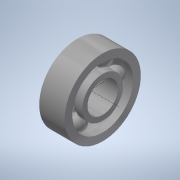
# Autodesk Inventor part: Ball bearing 15mm
Saved by Autodesk Inventor 2021 (Build 250183000, 183)
## iProperties
Manager: Pierloot J.
Company: Emmaüs Bovenbouw Aalter
Created: 2015-08-18
Part Number: Ball bearing 15mm
Material: S235
Catalog Web Link: http://emmausbovenbouw.op-weg.be/
Vendor: Emmaüsinstituut Bovenbouw Aalter
Document SubType Name: Modeling
Designer: Pierlootj
Engineer: Pierloot J.
Manufacturer: Standard
Standards Organization: Custom
Density: 7.86 g/cm^3
Appearance: Steel
Title: Algemene titel
Subject: Specifieke titel
Author: Pierlootj
Keywords: Ruwe Ø xxxxx
Comments: Opmerking
Autodesk Inventor part; units mm, degrees
ref_plane "YZ Plane" through (0, 0, 0) normal (1, 0, 0) x (0, 1, 0)
ref_plane "XZ Plane" through (0, 0, 0) normal (0, 1, 0) x (-1, 0, 0)
ref_plane "XY Plane" through (0, 0, 0) normal (0, 0, 1) x (1, 0, 0)
sketch "Sketch1" plane through (0, 0, 0) normal (0, 0, 1) x (1, 0, 0)
  line L0 (0, 2.8582) -> (0, -2.8582) construction
  line L1 (-5.7775, 0) -> (5.7775, 0) construction
  point P0 (0, 0)
  point P1 (0, 0)
  constraints: 4 end point, 2 midpoint, 1 coincident, 1 horizontal, 1 vertical
sketch "Sketch2" plane through (0, 0, 0) normal (0, 0, 1) x (1, 0, 0)
  line L0 (0, 0) -> (0, 7.5)
  line L1 (-2.5, 7.5) -> (2.5, 7.5)
  line L2 (2.5, 7.5) -> (2.5, 6)
  line L3 (2.5, 6) -> (-2.5, 6)
  line L4 (-2.5, 6) -> (-2.5, 7.5)
  line L5 (-2.5, 3) -> (2.5, 3)
  line L6 (2.5, 3) -> (2.5, 4)
  line L7 (2.5, 4) -> (-2.5, 4)
  line L8 (-2.5, 4) -> (-2.5, 3)
  line L9 (0, 4) -> (0, 5)
  circle A0 centre (0, 5) radius 1.5
  line L10 (-8.0884, 0) -> (8.0884, 0) projected
  point P0 (1.118, 4)
  point P1 (-1.118, 4)
  point P2 (-1.118, 6)
  point P3 (1.118, 6)
  dimension "d0" = 7.5
  dimension "d4" = 1.5
  dimension "d5" = 1
  dimension "d6" = 1
  dimension "d7" = 3
  constraints: 20 end point, 4 parallel, 2 horizontal, 2 perpendicular, 1 centre point, 1 coincident, 1 midpoint, 1 point on line, 1 vertical
  measures "d0" distance of L0.start L0.end
  measures "d4" distance of L1.end L2.end
  measures "d5" distance of L6.end L5.end
  measures "d6" distance of L9.start L9.end
  measures "d7" diameter of A0
revolve "Revolution1" add sketch "Sketch2" angle 360 about axis through (-10, 0, 0) along (1, 0, 0) contours A0 L7 L6 L5 L0 | L0 L5 L8 L7 A0 | L3 L4 L1 L0 A0 | L0 L1 L2 L3 A0
sketch "Sketch3" plane through (0, 0, 0) normal (0, 0, 1) x (1, 0, 0)
  line L0 (0, 0) -> (0, 7.5)
  line L1 (-2.5, 7.5) -> (2.5, 7.5)
  line L2 (2.5, 7.5) -> (2.5, 6)
  line L3 (-2.5, 6) -> (-2.5, 7.5)
  line L4 (-2.5, 3) -> (2.5, 3)
  line L5 (2.5, 3) -> (2.5, 4)
  line L6 (-2.5, 4) -> (-2.5, 3)
  line L7 (0, 4) -> (0, 5)
  circle A0 centre (0, 5) radius 1.5
  line L8 (-8.0884, 0) -> (8.0884, 0)
  line L9 (-1.5, 5) -> (1.5, 5)
  point P0 (1.118, 4)
  point P1 (-1.118, 4)
  point P2 (-1.118, 6)
  point P3 (1.118, 6)
  dimension "d9" = 7.5
  dimension "d10" = 1.5
  dimension "d11" = 1
  dimension "d12" = 1
  dimension "d13" = 3
  constraints: 20 end point, 3 horizontal, 2 parallel, 2 perpendicular, 2 point on circle, 1 centre point, 1 coincident, 1 point on line, 1 vertical
  measures "d9" distance of L0.start L0.end
  measures "d10" distance of L1.end L2.end
  measures "d11" distance of L5.end L4.end
  measures "d12" distance of L7.start L7.end
  measures "d13" diameter of A0
revolve "Revolution2" add sketch "Sketch3" angle 360 about axis through (-1.5, 5, 0) along (1, 0, 0) picked at (-0.8414, 5.5287) picked at (0.5287, 5.8414) contours L9 A0 L0 | L0 A0 L9
pattern_circular "Circular Pattern1" count 6 over 360 about axis through (-10, 0, 0) along (1, 0, 0) of "Revolution2"
body "Solid1"
